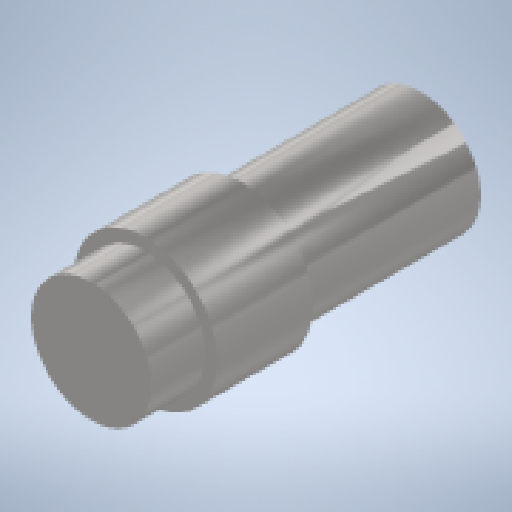
# Autodesk Inventor part: 出力ピン
Saved by Autodesk Inventor 2024 (Build 280153000, 153)
## iProperties
Created: 2023-05-29
Part Number: 出力ピン
Material: 鋼、炭素鋼
Document SubType Name: Modeling
Designer: yuta2
Density: 7.85 g/cm^3
Appearance: 半つや出し
Mass: 9.37137 g
Surface Area: 7.85398 cm^2
Volume: 1.19381 cm^3
Author: yuta2
Autodesk Inventor part; units mm, degrees
ref_plane "YZ Plane" through (0, 0, 0) normal (1, 0, 0) x (0, 1, 0)
ref_plane "XZ Plane" through (0, 0, 0) normal (0, 1, 0) x (-1, 0, 0)
ref_plane "XY Plane" through (0, 0, 0) normal (0, 0, 1) x (1, 0, 0)
sketch "スケッチ1" plane through (0, 0, 0) normal (1, 0, 0) x (0, 1, 0)
  line L0 (0, 0) -> (5, 0)
  line L1 (5, 0) -> (5, 4.5)
  line L2 (5, 4.5) -> (0, 4.5)
  line L3 (0, 4.5) -> (0, 0)
  line L4 (0, 0) -> (6, 0)
  line L5 (6, 0) -> (6, -8)
  line L6 (6, -8) -> (0, -8)
  line L7 (0, -8) -> (0, 0)
  line L8 (0, -8) -> (5, -8)
  line L9 (5, -8) -> (5, -23)
  line L10 (5, -23) -> (0, -23)
  line L11 (0, -23) -> (0, -8)
  point P0 (5, 0)
  dimension "d0" = 5
  dimension "d1" = 4.5
  dimension "d2" = 6
  dimension "d3" = 8
  dimension "d4" = 15
  constraints: 24 end point, 6 parallel, 3 horizontal, 3 perpendicular, 1 point on line
  measures "d0" distance of L2.end L1.end
  measures "d1" distance of L1.end L0.end
  measures "d2" distance of L5.end L6.end
  measures "d3" distance of L4.end L5.end
  measures "d4" distance of L8.end L9.end
revolve "回転1" add sketch "スケッチ1" angle 360 about axis through (0, 0, -23) along (0, 0, 1)
